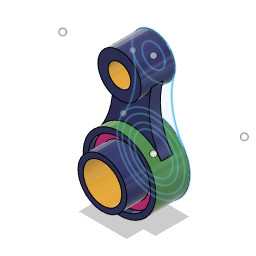
Questão5 (Autodesk Fusion 360 design; units mm, degrees)
Autodesk Fusion 360 part; units mm, degrees
sketch "Esboço1" plane through (0, 0, 0) normal (0, 0, 1) x (1, 0, 0)
  circle A0 centre (0, 75) radius 19
  circle A1 centre (0, 0) radius 32
  circle A2 centre (0, 75) radius 10
  circle A3 centre (0, 0) radius 17
  circle A4 centre (0, 0) radius 21.5
  circle A5 centre (0, 0) radius 27.5
  arc A6 (18.3212, 69.9669) -> (26.6783, 17.6711) centre (80.0349, 53.0133) ccw
  arc A7 (-26.6783, 17.6711) -> (-18.3212, 69.9669) centre (-80.0349, 53.0133) ccw
  dimension "d2" = 38
  dimension "d4" = 20
  dimension "d5" = 34
  dimension "d6" = 43
  dimension "d7" = 55
  dimension "d8" = 128
  constraint concentric A0 A2
  constraint concentric A1 A3
  constraint concentric A1 A4
  constraint concentric A1 A5
  constraint tangent A0 A6
  constraint tangent A1 A6
  constraint coincident A1 A6.end
  constraint coincident A0 A6.start
  measures "d2" diameter of A0
  measures "d4" diameter of A2
  measures "d5" diameter of A3
  measures "d6" diameter of A4
  measures "d7" diameter of A5
  measures "d8" diameter of A6
extrude "Extrusão1" add sketch "Esboço1" along normal blind 30 contours A0 makes body 1
extrude "Extrusão2" add sketch "Esboço1" along normal blind 30 separate body contours A1 makes body 2
extrude "Extrusão3" add sketch "Esboço1" along normal blind 25 contours A5 bodies 2
extrude "Extrusão4" add sketch "Esboço1" along normal blind 45 contours A4 bodies 2
extrude "Extrusão5" add sketch "Esboço1" along normal blind 20 contours A0 A1 A6 A7 bodies 1 2
extrude "Extrusão6" cut sketch "Esboço1" along normal blind 10 contours A0 A1 A6 A7 bodies 1
